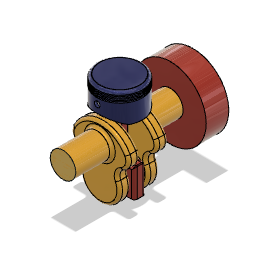
PISTON ASSEMBLY v3 (Autodesk Fusion 360 design; units mm, degrees)
Autodesk Fusion 360 part; units mm, degrees
sketch "Sketch1" plane through (0, 0, 0) normal (1, 0, 0) x (0, 0, -1)
  line L0 (0, 100) -> (0, 49)
  line L1 (0, 100) -> (40, 100)
  line L2 (40, 100) -> (40, 93)
  line L3 (40, 93) -> (36, 93)
  line L4 (36, 93) -> (36, 91)
  line L5 (36, 91) -> (40, 91)
  line L6 (40, 91) -> (40, 89)
  line L7 (40, 89) -> (36, 89)
  line L8 (36, 89) -> (36, 87)
  line L9 (36, 87) -> (40, 87)
  line L10 (40, 87) -> (40, 85)
  line L11 (40, 85) -> (36, 85)
  line L12 (36, 49) -> (0, 49)
  line L13 (0, 100) -> (0, 49)
  line L14 (36, 85) -> (36, 83)
  line L15 (36, 83) -> (40, 83)
  line L16 (40, 83) -> (40, 49)
  line L17 (36, 49) -> (40, 49)
  dimension "d1" = 40
  dimension "d2" = 7
  dimension "d3" = 4
  dimension "d4" = 2
  dimension "d5" = 36
  constraint vertical L0
  constraint perpendicular L0 L1
  constraint perpendicular L1 L2
  constraint perpendicular L2 L3
  constraint perpendicular L3 L4
  constraint perpendicular L4 L5
  constraint perpendicular L5 L6
  constraint perpendicular L6 L7
  constraint perpendicular L7 L8
  constraint perpendicular L8 L9
  constraint perpendicular L9 L10
  constraint perpendicular L10 L11
  constraint perpendicular L0 L12
  constraint perpendicular L11 L14
  constraint perpendicular L14 L15
  constraint perpendicular L15 L16
  constraint perpendicular L16 L17
  measures "d1" distance of L0.start L1.end
  measures "d2" distance of L1.end L2.end
  measures "d3" distance of L2.end L3.end
  measures "d4" distance of L3.end L4.end
  measures "d5" distance of L11.end L12.start
revolve "Revolve1" add sketch "Sketch1" angle 360 about axis through (0, 100, 0) along (0, -1, 0) makes body 1
sketch "Sketch2" plane through (0, 0, 0) normal (0, 0, 1) x (1, 0, 0)
  line L0 (0, 130) -> (0, 0)
  line L1 (-40, 49) -> (40, 49)
  arc A0 (35.5, 49) -> (-35.5, 49) centre (0, -9.0125) ccw
  line L2 (35.5, 49) -> (35.5, 35)
  line L3 (35.5, 35) -> (-35, 35)
  line L4 (-35, 35) -> (-35.5, 49)
  point P0 (0, 59)
  point P1 (-35.5, 49)
  point P2 (35.5, 49)
  dimension "d7" = 10
  dimension "d8" = 4.5
  constraint coincident L0.end origin
  constraint vertical L0
  constraint coincident L0 P0
  constraint coincident L1 P1
  constraint symmetric L0 P1 P2
  constraint coincident P0 A0
  constraint coincident P1 A0.end
  constraint coincident P2 A0.start
  constraint perpendicular L1 L2
  constraint perpendicular L2 L3
  measures "d7" distance of P0 L1
  measures "d8" distance of L1.start P1
sketch "Sketch3" plane through (0, 49, 0) normal (0, -1, 0) x (1, 0, 0)
  circle A0 centre (0, 0) radius 40
  circle A1 centre (0, 0) radius 35.5
  dimension "d9" = 71
  constraint coincident A0.centre A1.centre
  measures "d9" diameter of A1
extrude "Extrude1" cut sketch "Sketch3" against normal blind 50 contours A1 bodies 1
extrude "Extrude2" cut sketch "Sketch2" along normal mid plane 130 bodies 1
sketch "Sketch4" plane through (0, 0, 0) normal (0, 0, 1) x (1, 0, 0)
  circle A0 centre (0, 73) radius 5
  line L0 (35.5, 49) -> (40, 49)
  dimension "d14" = 10
  dimension "d15" = 24
  measures "d14" diameter of A0
  measures "d15" distance of A0.centre L0
extrude "Extrude3" cut sketch "Sketch4" along normal mid plane 120 bodies 1
fillet "Fillet1" radius 5 1 faces at (-6.4944, 100, -7.7208) on bodies 1
sketch "Sketch5" plane through (0, 0, 0) normal (0, 0, 1) x (1, 0, 0)
  spline S0 degree 3 poles (-5, 73) (-5, 73.6285) (-4.8743, 74.2985) (-4.3638, 75.5302) (-3.9791, 76.092) (-3.092, 76.9791) (-2.5302, 77.3638) (-1.2985, 77.8743) (-0.6285, 78) (0.6285, 78) (1.2985, 77.8743) (2.5302, 77.3638) (3.092, 76.9791) (3.9791, 76.092) (4.3638, 75.5302) (4.8743, 74.2985) (5, 73.6285) (5, 72.3715) (4.8743, 71.7015) (4.3638, 70.4698) (3.9791, 69.908) (3.092, 69.0209) (2.5302, 68.6362) (1.2985, 68.1257) (0.6285, 68) (-0.6285, 68) (-1.2985, 68.1257) (-2.5302, 68.6362) (-3.092, 69.0209) (-3.9791, 69.908) (-4.3638, 70.4698) (-4.8743, 71.7015) (-5, 72.3715) (-5, 73) knots 0 0 0 0 0.188556 0.188556 0.377112 0.377112 0.565667 0.565667 0.754221 0.754221 0.942775 0.942775 1.13133 1.13133 1.319886 1.319886 1.508442 1.508442 1.696998 1.696998 1.885554 1.885554 2.074108 2.074108 2.262663 2.262663 2.451217 2.451217 2.639772 2.639772 2.828328 2.828328 3.016884 3.016884 3.016884 3.016884
  spline S1 degree 3 poles (-5, 73) (-5, 72.3715) (-4.8743, 71.7015) (-4.3638, 70.4698) (-3.9791, 69.908) (-3.092, 69.0209) (-2.5302, 68.6362) (-1.2985, 68.1257) (-0.6285, 68) (0.6285, 68) (1.2985, 68.1257) (2.5302, 68.6362) (3.092, 69.0209) (3.9791, 69.908) (4.3638, 70.4698) (4.8743, 71.7015) (5, 72.3715) (5, 73.6285) (4.8743, 74.2985) (4.3638, 75.5302) (3.9791, 76.092) (3.092, 76.9791) (2.5302, 77.3638) (1.2985, 77.8743) (0.6285, 78) (-0.6285, 78) (-1.2985, 77.8743) (-2.5302, 77.3638) (-3.092, 76.9791) (-3.9791, 76.092) (-4.3638, 75.5302) (-4.8743, 74.2985) (-5, 73.6285) (-5, 73) knots 0 0 0 0 0.188556 0.188556 0.377112 0.377112 0.565667 0.565667 0.754221 0.754221 0.942775 0.942775 1.13133 1.13133 1.319886 1.319886 1.508442 1.508442 1.696998 1.696998 1.885554 1.885554 2.074108 2.074108 2.262663 2.262663 2.451217 2.451217 2.639772 2.639772 2.828328 2.828328 3.016884 3.016884 3.016884 3.016884
  spline S2 degree 3 poles (-35.5, 49) (-34.7819, 49.4395) (-33.9869, 49.9074) (-31.6722, 51.1984) (-30.0298, 52.0415) (-26.5489, 53.6333) (-24.584, 54.4424) (-20.2818, 55.9455) (-17.9443, 56.6386) (-13.0324, 57.7873) (-10.4532, 58.2434) (-5.2267, 58.8499) (-2.5793, 59) (2.5793, 59) (5.2267, 58.8499) (10.4532, 58.2434) (13.0324, 57.7873) (17.9443, 56.6386) (20.2818, 55.9455) (24.584, 54.4424) (26.5489, 53.6333) (30.0298, 52.0415) (31.6722, 51.1984) (33.9869, 49.9074) (34.7819, 49.4395) (35.5, 49) knots 14.292248 14.292248 14.292248 14.292248 14.751967 14.751967 15.530304 15.530304 16.304087 16.304087 17.077869 17.077869 17.851652 17.851652 18.625435 18.625435 19.399217 19.399217 20.173 20.173 20.946782 20.946782 21.720565 21.720565 22.498902 22.498902 22.958621 22.958621 22.958621 22.958621
  line L0 (35.5, 49) -> (40, 49)
  spline S3 degree 3 poles (35.5, 49) (34.7819, 49.4395) (33.9869, 49.9074) (31.6722, 51.1984) (30.0298, 52.0415) (26.5489, 53.6333) (24.584, 54.4424) (20.2818, 55.9455) (17.9443, 56.6386) (13.0324, 57.7873) (10.4532, 58.2434) (5.2267, 58.8499) (2.5793, 59) (-2.5793, 59) (-5.2267, 58.8499) (-10.4532, 58.2434) (-13.0324, 57.7873) (-17.9443, 56.6386) (-20.2818, 55.9455) (-24.584, 54.4424) (-26.5489, 53.6333) (-30.0298, 52.0415) (-31.6722, 51.1984) (-33.9869, 49.9074) (-34.7819, 49.4395) (-35.5, 49) knots 1.875291 1.875291 1.875291 1.875291 2.335011 2.335011 3.113348 3.113348 3.88713 3.88713 4.660913 4.660913 5.434696 5.434696 6.208478 6.208478 6.982261 6.982261 7.756043 7.756043 8.529826 8.529826 9.303609 9.303609 10.081945 10.081945 10.541665 10.541665 10.541665 10.541665
  line L1 (-40, 49) -> (-35.5, 49)
  line L2 (-40, 83) -> (40, 83)
  spline S4 degree 3 poles (-5, 73) (-5, 72.3715) (-4.8743, 71.7015) (-4.3638, 70.4698) (-3.9791, 69.908) (-3.092, 69.0209) (-2.5302, 68.6362) (-1.2985, 68.1257) (-0.6285, 68) (0.6285, 68) (1.2985, 68.1257) (2.5302, 68.6362) (3.092, 69.0209) (3.9791, 69.908) (4.3638, 70.4698) (4.8743, 71.7015) (5, 72.3715) (5, 73.6285) (4.8743, 74.2985) (4.3638, 75.5302) (3.9791, 76.092) (3.092, 76.9791) (2.5302, 77.3638) (1.2985, 77.8743) (0.6285, 78) (-0.6285, 78) (-1.2985, 77.8743) (-2.5302, 77.3638) (-3.092, 76.9791) (-3.9791, 76.092) (-4.3638, 75.5302) (-4.8743, 74.2985) (-5, 73.6285) (-5, 73) knots 0 0 0 0 0.188556 0.188556 0.377112 0.377112 0.565667 0.565667 0.754221 0.754221 0.942775 0.942775 1.13133 1.13133 1.319886 1.319886 1.508442 1.508442 1.696998 1.696998 1.885554 1.885554 2.074108 2.074108 2.262663 2.262663 2.451217 2.451217 2.639772 2.639772 2.828328 2.828328 3.016884 3.016884 3.016884 3.016884
  circle A0 centre (0, 73) radius 8.5
  line L3 (0, 73) -> (0, -47)
  circle A1 centre (0, -47) radius 23
  line L4 (-36, -22) -> (-36, -47)
  line L5 (0, -47) -> (-36, -47)
  line L6 (-8.5, 73.0024) -> (-8.5201, 2.9921)
  line L7 (-36, -22) -> (-33.5273, -22.0007)
  arc A2 (-33.5273, -22.0007) -> (-8.5201, 2.9921) centre (-33.5201, 2.9993) ccw
  line L8 (8.5, 73.0024) -> (8.5201, 2.9921)
  arc A3 (8.5201, 2.9921) -> (33.5273, -22.0007) centre (33.5201, 2.9993) ccw
  line L9 (36, -22) -> (33.5273, -22.0007)
  line L10 (36, -22) -> (36, -47)
  line L11 (0, -47) -> (36, -47)
  line L12 (36, -72) -> (36, -47)
  line L13 (-36, -72) -> (-36, -47)
  line L14 (36, -72) -> (-36, -72)
  arc A4 (-4.6, -12) -> (4.6, -12) centre (0, -12) ccw
  arc A5 (4.6, 58.0098) -> (-4.6, 58.0098) centre (0, 58) ccw
  line L15 (4.6, 58.8437) -> (4.6, -12)
  line L16 (-4.6, 73) -> (-4.6, 71.0404)
  line L17 (-4.6, 58.8437) -> (-4.6, -12)
  dimension "d19" = 17
  dimension "d20" = 120
  dimension "d21" = 46
  dimension "d22" = 36
  dimension "d23" = 25
  dimension "d24" = 25
  dimension "d26" = 9.2
  dimension "d27" = 15
  dimension "d28" = 9.2
  dimension "d29" = 35
  constraint coincident A0.centre L3.start
  constraint vertical L3
  constraint coincident L3.end A1.centre
  constraint vertical L4
  constraint perpendicular L3 L5
  constraint coincident A0 L6.start
  constraint tangent A0 L6
  constraint perpendicular L6 L7
  constraint tangent L6 A2
  constraint tangent L7 A2
  constraint symmetric L3 L4.start L9.start
  constraint symmetric L3 A1.centre L5.start
  constraint symmetric L3 L4.end L10.end
  constraint symmetric L3 L6.start L8.start
  constraint symmetric L3 L6.end L8.end
  constraint symmetric L3 L7.end A3.end
  constraint symmetric L3 A2 A3
  constraint symmetric L4.start L5 L13.start
  constraint symmetric L5 L4.end L13.end
  constraint symmetric L5 L9.start L12.start
  constraint symmetric L5 L10.end L11.end
  constraint coincident L3 A5.centre
  constraint coincident L3 A4.centre
  constraint parallel L3 L16
  constraint coincident A5.end L16
  constraint coincident S0 L16.end
  constraint collinear L16 L17
  constraint coincident S2 L15.start
  constraint coincident S2 L17.start
  measures "d19" diameter of A0
  measures "d20" distance of A0.centre L3.end
  measures "d21" diameter of A1
  measures "d22" distance of L3.end L4
  measures "d23" distance of L4.start L4.end
  measures "d24" radius of A2
  measures "d26" diameter of A5
  measures "d27" distance of A0.centre A5.centre
  measures "d28" diameter of A4
  measures "d29" distance of L3.end A4.centre
extrude "Extrude1'" add sketch "Sketch5" along normal mid plane 20 separate body contours S2 S3 A0 L3 L6 A5 | S2 S3 L3 A1 L4 L5 L6 L7 A2 A4 L17 | A0 L8 | S2 S3 A0 L3 L8 A5 | S2 S3 L3 A1 L8 A3 L9 L10 L11 A4 L15 | A1 L5 L11 L12 L13 L14 makes body 2 in component "Connecting rod"
sketch "Sketch6" plane through (0, 0, 0) normal (0, 0, 1) x (1, 0, 0)
  line L0 (0, -12) -> (0, -11)
  line L1 (-48.2521, -11.3402) -> (-54.9986, -11.3878)
  line L2 (47.7444, -10.6634) -> (54.9986, -10.6122)
  line L3 (23, -47) -> (28.802, -47)
  line L4 (23, -47) -> (22.9213, -35.839)
  arc A0 (54.9986, -10.6122) -> (-54.9986, -11.3878) centre (0, -11) ccw
  arc A1 (-31.9652, -32.7443) -> (31.761, -32.2949) centre (0, -47) ccw
  arc A2 (-42.0477, -12.0772) -> (-48.2521, -11.3402) centre (-48.0758, -36.3396) ccw
  arc A3 (47.7444, -10.6634) -> (41.5511, -11.4878) centre (47.9207, -35.6627) ccw
  circle A4 centre (-0.3878, 10) radius 22.5
  arc A5 (41.5511, -11.4878) -> (31.761, -32.2949) centre (45.3729, -25.9928) ccw
  arc A6 (-21.5395, -74.5871) -> (22.8067, -73.5491) centre (-0.7237, -16.0811) ccw
  arc A7 (-31.9652, -32.7443) -> (-42.0477, -12.0772) centre (-45.6646, -26.6346) ccw
  dimension "d33" = 36
  dimension "d35" = 25
  dimension "d36" = 45
  dimension "d37" = 22
  dimension "d52" = 35
  dimension "d53" = 15
  dimension "d54" = 15
  constraint vertical L0
  constraint horizontal L3
  constraint perpendicular L2 L4
  constraint tangent L1 A2
  constraint tangent L4 A3
  constraint tangent L2 A3
  constraint equal A2 A3
  constraint coincident L4.end A3
  constraint tangent A3 A5
  constraint tangent A1 A5
  constraint coincident A1 A6.start
  constraint coincident A1 A6.end
  constraint tangent A1 A7
  constraint tangent A2 A7
  measures "d33" distance of A1.centre L0.end
  measures "d35" radius of A2
  measures "d36" diameter of A4
  measures "d37" vertical distance of L0.start A4.centre
  measures "d52" radius of A1
  measures "d53" radius of A5
  measures "d54" radius of A7
extrude "Extrude4" add sketch "Sketch6" along normal blind 20 from surface at 15 separate body makes body 3
extrude "Extrude5" add 1 faces at (38.6176, 0.2468, 15) along direction (0, 0, -1) blind 20 from surface at 30 on bodies 3 bodies 3 makes body 4
sketch "Sketch7" plane through (0, 0, 0) normal (0, 0, 1) x (1, 0, 0)
  circle A0 centre (-0.3878, 10) radius 22.5
  circle A1 centre (-0.3878, 10) radius 22.5
  circle A2 centre (-0.3878, 10) radius 22.5
  circle A3 centre (-0.3878, 10) radius 22.5
  constraint concentric A1 A3
extrude "Extrude6" add sketch "Sketch7" along normal blind 60 bodies 3
delete_face "DeleteFace1" 1 faces at (-22.776, 12.2403, 5) on bodies 3
extrude "Extrude7" add 1 faces at (6.2185, 11.2399, 60) along direction (0, 0, 1) blind 40 on bodies 3 bodies 3
extrude "Extrude8" add 1 faces at (6.2185, 11.2399, 100) along direction (0, 0, 1) blind -190 and the other way blind 115 on bodies 3 bodies 3 4
sketch "Sketch8" plane through (0, 0, 0) normal (0, 0, 1) x (1, 0, 0)
  circle A0 centre (0, -47) radius 23
extrude "Extrude9" add sketch "Sketch8" along normal mid plane 40 bodies 3 4
fillet "Fillet2" radius 20 4 edges at (54.9986, -10.6122, 25) (54.9986, -10.6122, -25) (-54.9986, -11.3878, -25) (-54.9986, -11.3878, 25) on bodies 3 4
fillet "Fillet3" radius 5 4 faces at (38.1147, 15.8063, 35) (-22.6713, -0.999, -15) (-22.6713, -0.999, 15) (38.1147, 15.8063, -35) on bodies 3
fillet "Fillet1'" radius 5 16 edges at (36, -47, 10) (36, -47, -10) (34.7636, -22.0004, 10) (15.8475, -14.6835, 10) (8.5101, 37.9973, 10) (0, 81.5, 10) (-8.5101, 37.9973, 10) (-15.8475, -14.6835, 10) (-34.7636, -22.0004, 10) (-34.7636, -22.0004, -10) (-15.8475, -14.6835, -10) (-8.5101, 37.9973, -10) (0, 81.5, -10) (8.5101, 37.9973, -10) (15.8475, -14.6835, -10) (34.7636, -22.0004, -10) on bodies 2 in component "Connecting rod"
sketch "Sketch9" plane through (0, 0, 0) normal (0, 0, 1) x (1, 0, 0)
  spline S0 degree 3 poles (-5, 73) (-5, 73.6285) (-4.8743, 74.2985) (-4.3638, 75.5302) (-3.9791, 76.092) (-3.092, 76.9791) (-2.5302, 77.3638) (-1.2985, 77.8743) (-0.6285, 78) (0.6285, 78) (1.2985, 77.8743) (2.5302, 77.3638) (3.092, 76.9791) (3.9791, 76.092) (4.3638, 75.5302) (4.8743, 74.2985) (5, 73.6285) (5, 72.3715) (4.8743, 71.7015) (4.3638, 70.4698) (3.9791, 69.908) (3.092, 69.0209) (2.5302, 68.6362) (1.2985, 68.1257) (0.6285, 68) (-0.6285, 68) (-1.2985, 68.1257) (-2.5302, 68.6362) (-3.092, 69.0209) (-3.9791, 69.908) (-4.3638, 70.4698) (-4.8743, 71.7015) (-5, 72.3715) (-5, 73) knots 0 0 0 0 0.188556 0.188556 0.377112 0.377112 0.565667 0.565667 0.754221 0.754221 0.942775 0.942775 1.13133 1.13133 1.319886 1.319886 1.508442 1.508442 1.696998 1.696998 1.885554 1.885554 2.074108 2.074108 2.262663 2.262663 2.451217 2.451217 2.639772 2.639772 2.828328 2.828328 3.016884 3.016884 3.016884 3.016884
extrude "Extrude1''" add sketch "Sketch9" along normal mid plane 90 separate body makes body 5 in component "Component"
fillet "Fillet1''" radius 2.5 2 edges at (5, 73, 45) (5, 73, -45) on bodies 5 in component "Component"
sketch "Sketch10" plane through (0, 0, 100) normal (0, 0, 1) x (1, 0, 0)
  circle A0 centre (-0.3878, 10) radius 22.5
  circle A1 centre (-0.3878, 10) radius 54.2119
  constraint concentric A0 A1
sketch "Sketch11" plane through (0, 0, 100) normal (0, 0, 1) x (1, 0, 0)
  circle A0 centre (-0.3878, 10) radius 22.5
sketch "Sketch12" plane through (0, 0, 100) normal (0, 0, 1) x (1, 0, 0)
sketch "Sketch13" plane through (0, 0, -90) normal (0, 0, -1) x (-1, 0, 0)
  circle A0 centre (0.3878, 10) radius 22.5
  circle A1 centre (0.3878, 10) radius 63.2752
  circle A2 centre (0.3878, 10) radius 22.5
  constraint concentric A1 A2
extrude "Extrude10" add sketch "Sketch13" along normal blind 40 separate body makes body 6
copy_body "Body->Comp1" bodies 6 removing the originals makes body 7 in component "Component''"
component "Connecting rod" placed x (1, 0, 0) y (0, 1, 0) z (0, 0, 1) at (0, 0, 0)
component "Component" placed x (1, 0, 0) y (0, 1, 0) z (0, 0, 1) at (0, 0, 0)
component "Component'" placed x (1, 0, 0) y (0, 1, 0) z (0, 0, 1) at (0, 0, 0)
component "Component''" placed x (1, 0, 0) y (0, 1, 0) z (0, 0, 1) at (0, 0, 0)
equation "d9 = 35.5 * 2 mm"
named bodies: "PISTON", "crankshaft"
